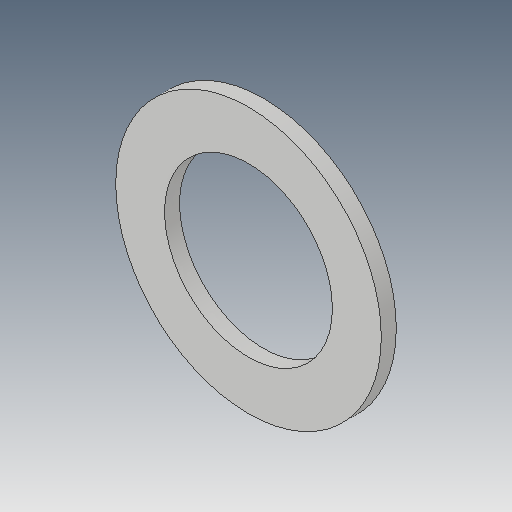
# Autodesk Inventor part: DelrinShim
Saved by Autodesk Inventor 2017 (Build 210142000, 142)
## iProperties
Created: 2016-08-14
Part Number: DelrinShim
Material: Generic
Document SubType Name: Modeling
Designer: User
Density: 1 g/cm^3
Appearance: Default
Mass: 0.0505733 g
Surface Area: 1.88903 cm^2
Volume: 0.0505733 cm^3
Author: User
Autodesk Inventor part; units mm, degrees
ref_plane "YZ Plane" through (0, 0, 0) normal (1, 0, 0) x (0, 1, 0)
ref_plane "XZ Plane" through (0, 0, 0) normal (0, 1, 0) x (-1, 0, 0)
ref_plane "XY Plane" through (0, 0, 0) normal (0, 0, 1) x (1, 0, 0)
sketch "Sketch1" plane through (0, 0, 0) normal (0, 0, 1) x (1, 0, 0)
  circle A0 centre (7.7, 0) radius 3.9095
  circle A1 centre (7.7, 0) radius 6.1872
  point P0 (0, 0)
  constraints: 2 centre point, 1 coincident, 2 other
extrude "Extrusion1" add sketch "Sketch1" along normal blind 0.7
body "Solid1"
